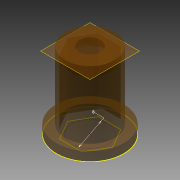
# Autodesk Inventor part: z-keeper
Saved by Autodesk Inventor 2014 (Build 180170000, 170)
## iProperties
Created: 2014-01-09
Part Number: z-keeper
Material: Generic
Document SubType Name: Modeling
Designer: caleb
Density: 1 g/cm^3
Appearance: Polycarbonate - Smoked
Author: caleb
Autodesk Inventor part; units mm, degrees
ref_plane "YZ Plane" through (0, 0, 0) normal (1, 0, 0) x (0, 1, 0)
ref_plane "XZ Plane" through (0, 0, 0) normal (0, 1, 0) x (-1, 0, 0)
ref_plane "XY Plane" through (0, 0, 0) normal (0, 0, 1) x (1, 0, 0)
sketch "Sketch2" plane through (0, 0, 0) normal (0, 0, 1) x (1, 0, 0)
  circle A0 centre (0, 0) radius 7.5
  dimension "d0" = 15
  constraints: 1 centre point, 1 coincident
  measures "d0" diameter of A0
extrude "Extrusion1" add sketch "Sketch2" along normal blind 2
sketch "Sketch3" plane through (0, 0, 2) normal (0, 0, 1) x (1, 0, 0)
  circle A0 centre (0, 0) radius 7.5 projected
  circle A1 centre (0, 0) radius 5.5
  dimension "d3" = 11
  constraints: 1 centre point, 1 coincident
  measures "d3" diameter of A1
extrude "Extrusion2" add sketch "Sketch3" along normal blind 15 contours A1
sketch "Sketch4" plane through (0, 0, 0) normal (0, 0, -1) x (-1, 0, 0)
  circle A0 centre (0, 0) radius 7.5 projected
  constraints: 1 coincident
hole "Hole1" at (0, 0, 0) direction (0, 0, 1) diameter 4.7 end through all
ref_plane "Work Plane1" through (0, 0, 16) normal (0, 0, 1) x (1, 0, 0)
sketch "Sketch5" plane through (0, 0, 0) normal (0, 0, -1) x (-1, 0, 0)
  circle A0 centre (0, 0) radius 2.35 projected
  circle A1 centre (0, 0) radius 7.5 projected
  line L0 (2.4934, 4.3187) -> (4.9869, 0)
  line L1 (4.9869, 0) -> (2.4934, -4.3188)
  line L2 (2.4934, -4.3188) -> (-2.4934, -4.3187)
  line L3 (-2.4934, -4.3187) -> (-4.9869, 0)
  line L4 (-4.9869, 0) -> (-2.4934, 4.3187)
  line L5 (-2.4934, 4.3187) -> (2.4934, 4.3187)
  dimension "d14" = 8.6375
  constraints: 12 end point, 1 coincident, 1 horizontal, 13 other
  measures "d14" distance between parallel lines of L2 L5
extrude "Extrusion3" cut sketch "Sketch5" against normal up to surface (16 mm away) contours L0 L1 L2 L3 L4 L5
sketch "Sketch6" plane through (0, 0, 0) normal (0, 0, -1) x (-1, 0, 0)
  line L0 (2.4934, -4.3188) -> (-2.4934, -4.3187) projected
  line L1 (-2.4934, -4.3187) -> (-4.9869, 0) projected
  line L2 (-4.9869, 0) -> (-2.4934, 4.3187) projected
  line L3 (-2.4934, 4.3187) -> (2.4934, 4.3187) projected
  line L4 (2.4934, 4.3187) -> (4.9869, 0) projected
  line L5 (4.9869, 0) -> (2.4934, -4.3188) projected
  circle A0 centre (0, 0) radius 7.5 projected
  circle A1 centre (0, 0) radius 4 construction
  dimension "d17" = 8
  constraints: 1 centre point, 1 coincident
  measures "d17" diameter of A1
sketch "Sketch7" plane through (0, 0, 0) normal (1, 0, 0) x (0, 1, 0)
  line L0 (-7.5, 0) -> (-7.5, 2) projected
  line L1 (-7.5, 2) -> (-5.5, 2) projected
  line L2 (-5.5, 2) -> (-5.5, 17) projected
  line L3 (-5.5, 17) -> (-2.35, 17) projected
  line L4 (-2.35, 17) -> (-2.35, 16) projected
  line L5 (-2.35, 16) -> (-4.3187, 16) projected
  line L6 (-4.3187, 16) -> (-4.3187, 0) projected
  line L7 (-4.3187, 0) -> (-7.5, 0) projected
  line L8 (7.5, 2) -> (7.5, 0) projected
  line L9 (7.5, 0) -> (4.3187, 0) projected
  line L10 (4.3187, 0) -> (4.3187, 16) projected
  line L11 (4.3187, 16) -> (2.35, 16) projected
  line L12 (2.35, 16) -> (2.35, 17) projected
  line L13 (2.35, 17) -> (5.5, 17) projected
  line L14 (5.5, 17) -> (5.5, 2) projected
  line L15 (5.5, 2) -> (7.5, 2) projected
  line L16 (2.35, 16) -> (4.3187, 14.0313)
  line L17 (0, -3.4) -> (0, 20.4) projected
  point P0 (0, 0)
  dimension "d18" = 45
  constraints: 2 end point, 1 point on line
  measures "d18" angle of L10 L16
revolve "Revolution1" add sketch "Sketch7" angle 360 about axis through (0, 0, -10) along (0, 0, 1) contours L16 L11 L10
chamfer "Chamfer1" distance 2 angle 45 6 edges at (0, -4.3187, 0) (3.7401, -2.1594, 0) (3.7401, 2.1594, 0) (0, 4.3187, 0) (-3.7401, 2.1594, 0) (-3.7401, -2.1594, 0)
body "Solid1"
